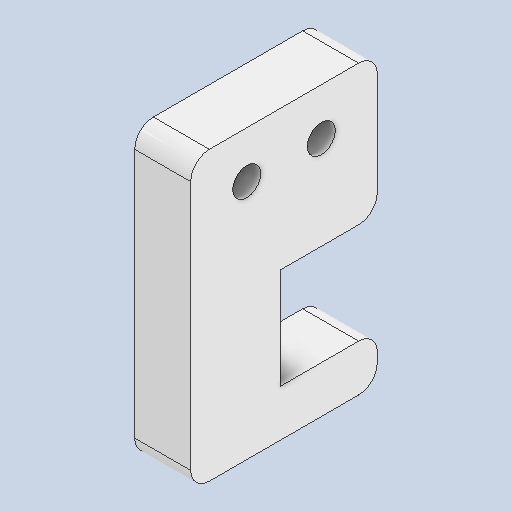
# Autodesk Inventor part: base_weel-v2-POM-pc-F-2
Saved by Autodesk Inventor 2025.2 (Build 292293000, 293)
## iProperties
Created: 2025-01-14
Part Number: base_weel-v2-POM-pc-F-2
Material: ABS プラスチック
Document SubType Name: Modeling
Designer: haruy
Density: 1.06 g/cm^3
Appearance: 白
Author: haruy
Autodesk Inventor part; units mm, degrees
ref_plane "YZ Plane" through (0, 0, 0) normal (1, 0, 0) x (0, 1, 0)
ref_plane "XZ Plane" through (0, 0, 0) normal (0, 1, 0) x (-1, 0, 0)
ref_plane "XY Plane" through (0, 0, 0) normal (0, 0, 1) x (1, 0, 0)
sketch "スケッチ1" plane through (0, 0, 0) normal (1, 0, 0) x (0, 1, 0)
  line L0 (0, 0) -> (10, 0)
  line L1 (10, 0) -> (10, -61.0895)
  line L2 (10, -61.0895) -> (0, -61.0895)
  line L3 (0, -61.0895) -> (0, 0)
  line L4 (10, 0) -> (-20.8, 0)
  line L5 (-20.8, 0) -> (-20.8, -20)
  line L6 (-20.8, -20) -> (10, -20)
  line L7 (10, -20) -> (10, 0)
  line L8 (-15.8, -20) -> (-5, -20)
  line L9 (-5, -20) -> (-5, -9.6)
  line L10 (-5, -9.6) -> (-15.8, -9.6)
  line L11 (-15.8, -9.6) -> (-15.8, -20)
  circle A0 centre (5, -6) radius 1.5
  circle A1 centre (5, -14) radius 1.5
  point P0 (-5.4, -20)
  dimension "d0" = 10
  dimension "d2" = 20
  dimension "d4" = 10.4
  dimension "d5" = 5
  dimension "d6" = 3
  dimension "d7" = 3
  dimension "d8" = 6
  dimension "d9" = 8
  dimension "d10" = 5
  dimension "d11" = 5
  dimension "d14" = 5
  dimension "d15" = 10.8
  constraints: 24 end point, 6 parallel, 3 horizontal, 3 perpendicular, 2 centre point, 1 midpoint, 1 point on line
  measures "d0" distance of L1.end L2.end
  measures "d2" distance from line of L4 point (-5.4, -20)
  measures "d4" distance of L9.end L8.end
  measures "d5" distance between parallel lines of L5 L11
  measures "d6" diameter of A0
  measures "d7" diameter of A1
  measures "d8" distance from line of A0.centre L0
  measures "d9" distance of A1.centre A0.centre
  measures "d10" distance from line of A0.centre L1
  measures "d11" distance from line of A1.centre L7
  measures "d14" distance between parallel lines of L3 L9
  measures "d15" distance between parallel lines of L11 L9
extrude "押し出し1" add sketch "スケッチ1" along normal blind 6 contours L0 L1 L6 L3 | L3 L6 L9 L10 L11 L5 L4
fillet "フィレット1" radius 2 6 edges at (3, 10, -20) (3, 10, 0) (3, -20.8, 0) (3, -20.8, -20) (3, -5, -20) (3, -15.8, -20)
sketch "スケッチ2" plane through (6, 0, 0) normal (1, 0, 0) x (0, 0, -1)
  arc A0 (20, -17.8) -> (18, -15.8) centre (18, -17.8) ccw projected
  line L0 (18, -15.8) -> (9.6, -15.8) projected
  line L1 (9.6, -15.8) -> (9.6, -5) projected
  line L2 (9.6, -5) -> (18, -5) projected
  arc A1 (18, -5) -> (20, -3) centre (18, -3) ccw projected
  line L3 (20, -3) -> (20, 8) projected
  arc A2 (20, 8) -> (18, 10) centre (18, 8) ccw projected
  line L4 (18, 10) -> (2, 10) projected
  arc A3 (2, 10) -> (0, 8) centre (2, 8) ccw projected
  line L5 (0, 8) -> (0, -18.8) projected
  arc A4 (0, -18.8) -> (2, -20.8) centre (2, -18.8) ccw projected
  line L6 (2, -20.8) -> (18, -20.8) projected
  arc A5 (18, -20.8) -> (20, -18.8) centre (18, -18.8) ccw projected
  line L7 (20, -18.8) -> (20, -17.8) projected
  circle A6 centre (6, 5) radius 1.5 projected
  circle A7 centre (14, 5) radius 1.5 projected
  point P0 (0, 0)
equation "\"d11\" = d10"
